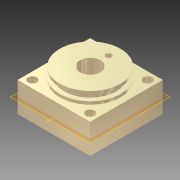
# Autodesk Inventor part: TU-002
Saved by Autodesk Inventor 2011 (Build 150229000, 229)
## iProperties
Created: 2008-05-12
Part Number: TU-002
Document SubType Name: Modeling
Designer: PN
Density: 7.86 g/cm^3
Material: Steel, Mild
Description: Cylinder Head Cover_Front
Mass: 394.415 g
Surface Area: 129.648 cm^2
Volume: 50.1801 cm^3
Author: PN
Autodesk Inventor part; units mm, degrees
ref_plane "YZ Plane" through (0, 0, 0) normal (1, 0, 0) x (0, 1, 0)
ref_plane "XZ Plane" through (0, 0, 0) normal (0, 1, 0) x (-1, 0, 0)
ref_plane "XY Plane" through (0, 0, 0) normal (0, 0, 1) x (1, 0, 0)
sketch "Sketch1" plane through (0, 0, 0) normal (0, 0, 1) x (1, 0, 0)
  line L0 (-24.5, 24.5) -> (24.5, 24.5)
  line L1 (24.5, 24.5) -> (24.5, -24.5)
  line L2 (24.5, -24.5) -> (-24.5, -24.5)
  line L3 (-24.5, -24.5) -> (-24.5, 24.5)
  point P0 (0, 0)
  point P1 (-24.5, 0)
  point P2 (0, 24.5)
  dimension "Width" = 49
  dimension "Height" = 49
  constraints: 8 end point, 2 midpoint, 2 parallel, 1 horizontal, 1 horizontal alignment, 1 perpendicular, 1 vertical alignment
  measures "Width" distance of L0.start L0.end
  measures "Height" distance of L2.end L0.start
extrude "Extrusion1" add sketch "Sketch1" along normal blind 20
sketch "Sketch2" plane through (0, 0, 20) normal (0, 0, 1) x (1, 0, 0)
  line L0 (24.5, 24.5) -> (24.5, -24.5) projected
  line L1 (-24.5, 24.5) -> (24.5, 24.5) projected
  line L2 (-24.5, -24.5) -> (-24.5, 24.5) projected
  line L3 (24.5, -24.5) -> (-24.5, -24.5) projected
  line L4 (19.5, 19.5) -> (19.5, -19.5)
  line L5 (19.5, -19.5) -> (-19.5, -19.5)
  line L6 (-19.5, -19.5) -> (-19.5, 19.5)
  line L7 (-19.5, 19.5) -> (19.5, 19.5)
  point P0 (0, 0)
  dimension "d4" = 5
  dimension "d5" = 39
  dimension "d6" = 39
  constraints: 8 end point, 3 other
  measures "d4" distance between parallel lines of L6 L2
  measures "d5" distance of L4.end L5.end
  measures "d6" distance of L5.end L6.end
hole "Hole1" at (-19.5, -19.5, 20) direction (0, 0, -1) diameter 6 end through all
pattern_linear "Rectangular Pattern1" count 2 spacing 39 along (1, 0, 0) count 2 spacing 39 along (0, 1, 0) of "Hole1"
sketch "Sketch3" plane through (0, 0, 0) normal (1, 0, 0) x (0, 1, 0)
  line L0 (-24.5, 20) -> (24.5, 20) projected
  line L1 (0, 20) -> (0, 28)
  line L2 (0, 28) -> (20.5, 28)
  line L3 (20.5, 28) -> (20.5, 26)
  line L4 (20.5, 26) -> (17.5, 26)
  line L5 (17.5, 26) -> (17.5, 22)
  line L6 (17.5, 22) -> (20.5, 22)
  line L7 (20.5, 22) -> (20.5, 20)
  point P0 (0, 0)
  dimension "d25" = 8
  dimension "d26" = 20.5
  dimension "d27" = 2
  dimension "d28" = 4
  dimension "d29" = 17.5
  constraints: 14 end point, 4 perpendicular, 2 collinear, 2 parallel, 1 midpoint, 1 point on line
  measures "d25" distance of L1.start L1.end
  measures "d26" distance of L1.end L2.end
  measures "d27" distance of L2.end L3.end
  measures "d28" distance of L4.end L5.end
  measures "d29" distance between parallel lines of L5 L1
revolve "Revolution1" add sketch "Sketch3" angle 360 about axis through (0, 0, 20) along (0, 0, 1)
sketch "Sketch4" plane through (-24.5, 24.5, 0) normal (0, 1, 0) x (1, 0, 0)
  line L0 (0, -20) -> (49, -20) projected
  line L1 (0, 0) -> (0, -20) projected
  line L2 (24.5, -20) -> (24.5, -10)
  point P0 (24.5, 0)
  dimension "d31" = 10
  constraints: 2 end point, 1 midpoint, 1 parallel
  measures "d31" distance of L2.start L2.end
hole "Hole4" at (0, 24.5, 10) direction (0, -1, 0) diameter 4.134 depth 14 tip angle 118 thread size "M5x0.8" class "6H" standard "ANSI Metric M Profile"
ref_plane "Work Plane3" through (0, 24.5, 10) normal (0, 0, 1) x (0, -1, 0)
sketch "Sketch7" plane through (0, 0, 28) normal (0, 0, 1) x (1, 0, 0)
  circle A0 centre (0, 0) radius 20.5 projected
  line L0 (0, 0) -> (0, 12.5)
  dimension "d56" = 12.5
  constraints: 2 end point, 1 coincident, 1 vertical
  measures "d56" distance of L0.start L0.end
hole "Hole5" at (0, 12.5, 28) direction (0, 0, -1) diameter 4 depth 18
hole "Hole6" at (0, 0, 28) direction (0, 0, -1) diameter 14 end through all
equation "\"Height\" = Width"
equation "\"d16\" = d5"
equation "\"d19\" = d6"
body "Solid1"
